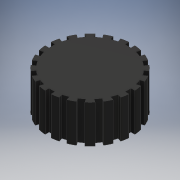
# Autodesk Inventor part: Llanta
Saved by Autodesk Inventor 2017 (Build 210142000, 142)
## iProperties
Part Number: Llanta
Material: Goma
Document SubType Name: Modeling
Designer: fam
Density: 0.93 g/cm^3
Appearance: Goma - Negro
Author: fam
Autodesk Inventor part; units mm, degrees
ref_plane "YZ Plane" through (0, 0, 0) normal (1, 0, 0) x (0, 1, 0)
ref_plane "XZ Plane" through (0, 0, 0) normal (0, 1, 0) x (-1, 0, 0)
ref_plane "XY Plane" through (0, 0, 0) normal (0, 0, 1) x (1, 0, 0)
sketch "Boceto1" plane through (0, 0, 0) normal (0, 0, 1) x (1, 0, 0)
  circle A0 centre (0, 0) radius 21
  dimension "d0" = 42
  constraints: 1 centre point, 1 coincident
  measures "d0" diameter of A0
extrude "Extrusión1" add sketch "Boceto1" along normal blind 19
sketch "Boceto2" plane through (0, 0, 19) normal (0, 0, 1) x (1, 0, 0)
  circle A0 centre (0, 0) radius 21 construction
  circle A1 centre (0, 0) radius 21 projected
  circle A2 centre (0, 0) radius 19 construction
  arc A3 (1.5, 20.9464) -> (-1.5, 20.9464) centre (0, 0) ccw
  line L0 (1.5, 20.9464) -> (1.5, 18.9407)
  line L1 (-1.5, 20.9464) -> (-1.5, 18.9407)
  arc A4 (1.5, 18.9407) -> (-1.5, 18.9407) centre (0, 0) ccw
  arc A5 (7.8994, 19.4576) -> (5.0462, 20.3847) centre (0, 0) ccw
  line L2 (7.8994, 19.4576) -> (7.2796, 17.5501)
  line L3 (5.0462, 20.3847) -> (4.4264, 18.4772)
  arc A6 (7.2796, 17.5501) -> (4.4264, 18.4772) centre (0, 0) ccw
  arc A7 (13.5255, 16.0643) -> (11.0984, 17.8276) centre (0, 0) ccw
  line L4 (13.5255, 16.0643) -> (12.3466, 14.4417)
  line L5 (11.0984, 17.8276) -> (9.9195, 16.205)
  arc A8 (12.3466, 14.4417) -> (9.9195, 16.205) centre (0, 0) ccw
  arc A9 (17.8276, 11.0984) -> (16.0643, 13.5255) centre (0, 0) ccw
  line L6 (17.8276, 11.0984) -> (16.205, 9.9195)
  line L7 (16.0643, 13.5255) -> (14.4417, 12.3466)
  arc A10 (16.205, 9.9195) -> (14.4417, 12.3466) centre (0, 0) ccw
  arc A11 (20.3847, 5.0462) -> (19.4576, 7.8994) centre (0, 0) ccw
  line L8 (20.3847, 5.0462) -> (18.4772, 4.4264)
  line L9 (19.4576, 7.8994) -> (17.5501, 7.2796)
  arc A12 (18.4772, 4.4264) -> (17.5501, 7.2796) centre (0, 0) ccw
  arc A13 (20.9464, -1.5) -> (20.9464, 1.5) centre (0, 0) ccw
  line L10 (20.9464, -1.5) -> (18.9407, -1.5)
  line L11 (20.9464, 1.5) -> (18.9407, 1.5)
  arc A14 (18.9407, -1.5) -> (18.9407, 1.5) centre (0, 0) ccw
  arc A15 (19.4576, -7.8994) -> (20.3847, -5.0462) centre (0, 0) ccw
  line L12 (19.4576, -7.8994) -> (17.5501, -7.2796)
  line L13 (20.3847, -5.0462) -> (18.4772, -4.4264)
  arc A16 (17.5501, -7.2796) -> (18.4772, -4.4264) centre (0, 0) ccw
  arc A17 (16.0643, -13.5255) -> (17.8276, -11.0984) centre (0, 0) ccw
  line L14 (16.0643, -13.5255) -> (14.4417, -12.3466)
  line L15 (17.8276, -11.0984) -> (16.205, -9.9195)
  arc A18 (14.4417, -12.3466) -> (16.205, -9.9195) centre (0, 0) ccw
  arc A19 (11.0984, -17.8276) -> (13.5255, -16.0643) centre (0, 0) ccw
  line L16 (11.0984, -17.8276) -> (9.9195, -16.205)
  line L17 (13.5255, -16.0643) -> (12.3466, -14.4417)
  arc A20 (9.9195, -16.205) -> (12.3466, -14.4417) centre (0, 0) ccw
  arc A21 (5.0462, -20.3847) -> (7.8994, -19.4576) centre (0, 0) ccw
  line L18 (5.0462, -20.3847) -> (4.4264, -18.4772)
  line L19 (7.8994, -19.4576) -> (7.2796, -17.5501)
  arc A22 (4.4264, -18.4772) -> (7.2796, -17.5501) centre (0, 0) ccw
  arc A23 (-1.5, -20.9464) -> (1.5, -20.9464) centre (0, 0) ccw
  line L20 (-1.5, -20.9464) -> (-1.5, -18.9407)
  line L21 (1.5, -20.9464) -> (1.5, -18.9407)
  arc A24 (-1.5, -18.9407) -> (1.5, -18.9407) centre (0, 0) ccw
  arc A25 (-7.8994, -19.4576) -> (-5.0462, -20.3847) centre (0, 0) ccw
  line L22 (-7.8994, -19.4576) -> (-7.2796, -17.5501)
  line L23 (-5.0462, -20.3847) -> (-4.4264, -18.4772)
  arc A26 (-7.2796, -17.5501) -> (-4.4264, -18.4772) centre (0, 0) ccw
  arc A27 (-13.5255, -16.0643) -> (-11.0984, -17.8276) centre (0, 0) ccw
  line L24 (-13.5255, -16.0643) -> (-12.3466, -14.4417)
  line L25 (-11.0984, -17.8276) -> (-9.9195, -16.205)
  arc A28 (-12.3466, -14.4417) -> (-9.9195, -16.205) centre (0, 0) ccw
  arc A29 (-17.8276, -11.0984) -> (-16.0643, -13.5255) centre (0, 0) ccw
  line L26 (-17.8276, -11.0984) -> (-16.205, -9.9195)
  line L27 (-16.0643, -13.5255) -> (-14.4417, -12.3466)
  arc A30 (-16.205, -9.9195) -> (-14.4417, -12.3466) centre (0, 0) ccw
  arc A31 (-20.3847, -5.0462) -> (-19.4576, -7.8994) centre (0, 0) ccw
  line L28 (-20.3847, -5.0462) -> (-18.4772, -4.4264)
  line L29 (-19.4576, -7.8994) -> (-17.5501, -7.2796)
  arc A32 (-18.4772, -4.4264) -> (-17.5501, -7.2796) centre (0, 0) ccw
  arc A33 (-20.9464, 1.5) -> (-20.9464, -1.5) centre (0, 0) ccw
  line L30 (-20.9464, 1.5) -> (-18.9407, 1.5)
  line L31 (-20.9464, -1.5) -> (-18.9407, -1.5)
  arc A34 (-18.9407, 1.5) -> (-18.9407, -1.5) centre (0, 0) ccw
  arc A35 (-19.4576, 7.8994) -> (-20.3847, 5.0462) centre (0, 0) ccw
  line L32 (-19.4576, 7.8994) -> (-17.5501, 7.2796)
  line L33 (-20.3847, 5.0462) -> (-18.4772, 4.4264)
  arc A36 (-17.5501, 7.2796) -> (-18.4772, 4.4264) centre (0, 0) ccw
  arc A37 (-16.0643, 13.5255) -> (-17.8276, 11.0984) centre (0, 0) ccw
  line L34 (-16.0643, 13.5255) -> (-14.4417, 12.3466)
  line L35 (-17.8276, 11.0984) -> (-16.205, 9.9195)
  arc A38 (-14.4417, 12.3466) -> (-16.205, 9.9195) centre (0, 0) ccw
  arc A39 (-11.0984, 17.8276) -> (-13.5255, 16.0643) centre (0, 0) ccw
  line L36 (-11.0984, 17.8276) -> (-9.9195, 16.205)
  line L37 (-13.5255, 16.0643) -> (-12.3466, 14.4417)
  arc A40 (-9.9195, 16.205) -> (-12.3466, 14.4417) centre (0, 0) ccw
  arc A41 (-5.0462, 20.3847) -> (-7.8994, 19.4576) centre (0, 0) ccw
  line L38 (-5.0462, 20.3847) -> (-4.4264, 18.4772)
  line L39 (-7.8994, 19.4576) -> (-7.2796, 17.5501)
  arc A42 (-4.4264, 18.4772) -> (-7.2796, 17.5501) centre (0, 0) ccw
  point P0 (0, 21)
  point P1 (6.4894, 19.9722)
  point P2 (12.3435, 16.9894)
  point P3 (16.9894, 12.3435)
  point P4 (19.9722, 6.4894)
  point P5 (21, 0)
  point P6 (19.9722, -6.4894)
  point P7 (16.9894, -12.3435)
  point P8 (12.3435, -16.9894)
  point P9 (6.4894, -19.9722)
  point P10 (0, -21)
  point P11 (-6.4894, -19.9722)
  point P12 (-12.3435, -16.9894)
  point P13 (-16.9894, -12.3435)
  point P14 (-19.9722, -6.4894)
  point P15 (-21, 0)
  point P16 (-19.9722, 6.4894)
  point P17 (-16.9894, 12.3435)
  point P18 (-12.3435, 16.9894)
  point P19 (-6.4894, 19.9722)
  dimension "d3" = 38
  dimension "d4" = 3
  dimension "d7" = 360
  constraints: 83 point on circle, 80 end point, 42 centre point, 6 concentric, 2 vertical, 1 vertical alignment, 221 other
  measures "d3" diameter of A2
  measures "d4" distance of L0.start L1.start
extrude "Extrusión2" cut sketch "Boceto2" against normal through all contours A1 L10 A14 L11 | L8 A12 L9 A1 | A1 L12 A16 L13 | L6 A10 L7 A1 | A1 L14 A18 L15 | L4 A8 L5 A1 | A1 L16 A20 L17 | L2 A6 L3 A1 | A1 L18 A22 L19 | L0 A4 L1 A1 | A1 L20 A24 L21 | L38 A42 L39 A1 | A1 L22 A26 L23 | L36 A40 L37 A1 | A1 L24 A28 L25 | L34 A38 L35 A1 | A1 L26 A30 L27 | L32 A36 L33 A1 | A1 L28 A32 L29 | L30 A34 L31 A1
